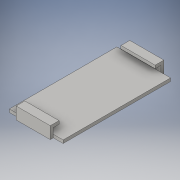
# Autodesk Inventor part: PanelHolder
Saved by Autodesk Inventor 2016 (Build 200138000, 138)
## iProperties
Created: 2016-08-20
Part Number: PanelHolder
Material: Generic
Document SubType Name: Modeling
Designer: yash
Density: 1 g/cm^3
Appearance: Default
Author: yash
Autodesk Inventor part; units mm, degrees
ref_plane "YZ Plane" through (0, 0, 0) normal (1, 0, 0) x (0, 1, 0)
ref_plane "XZ Plane" through (0, 0, 0) normal (0, 1, 0) x (-1, 0, 0)
ref_plane "XY Plane" through (0, 0, 0) normal (0, 0, 1) x (1, 0, 0)
sketch "Sketch1" plane through (0, 0, 0) normal (0, 1, 0) x (-1, 0, 0)
  line L0 (0, 0) -> (30, 0)
  line L1 (30, 0) -> (30, -60)
  line L2 (30, -60) -> (0, -60)
  line L3 (0, -60) -> (0, 0)
  dimension "d0" = 30
  dimension "d1" = 60
  constraints: 8 end point, 2 parallel, 1 horizontal, 1 perpendicular
  measures "d0" distance of L1.end L2.end
  measures "d1" distance of L0.end L1.end
extrude "Extrusion1" add sketch "Sketch1" along normal blind 1.7272
sketch "Sketch2" plane through (-30, 0, 0) normal (0, 0, 1) x (1, 0, 0)
  line L0 (30, 0) -> (0, 0) projected
  line L1 (5.475, 0) -> (24.525, 0)
  line L2 (24.525, 0) -> (24.525, 6.7272)
  line L3 (24.525, 6.7272) -> (5.475, 6.7272)
  line L4 (5.475, 6.7272) -> (5.475, 0)
  point P0 (15, 6.7272)
  point P1 (15, 0)
  dimension "d4" = 19.05
  dimension "d5" = 6.7272
  constraints: 8 end point, 2 midpoint, 2 parallel, 1 horizontal, 1 perpendicular, 1 point on line, 1 vertical alignment
  measures "d4" distance of L3.end L2.end
  measures "d5" distance of L2.end L1.end
extrude "Extrusion2" add sketch "Sketch2" along normal blind 1.7272
sketch "Sketch3" plane through (-30, 0, 0) normal (0, 0, -1) x (-1, 0, 0)
  line L0 (-24.525, 6.7272) -> (-5.475, 6.7272) projected
  line L1 (-5.475, 6.7272) -> (-5.475, 1.7272) projected
  line L2 (-24.525, 6.7272) -> (-5.475, 6.7272)
  line L3 (-5.475, 6.7272) -> (-5.475, 5)
  line L4 (-5.475, 5) -> (-24.525, 5)
  line L5 (-24.525, 5) -> (-24.525, 6.7272)
  point P0 (-30, 0)
  dimension "d8" = 1.7272
  constraints: 8 end point, 2 parallel, 1 horizontal, 1 perpendicular, 1 point on line
  measures "d8" distance of L2.end L3.end
extrude "Extrusion3" add sketch "Sketch3" along normal blind 3.175
sketch "Sketch4" plane through (0, 0, -60) normal (0, 0, -1) x (-1, 0, 0)
  line L0 (30, 0) -> (0, 0) projected
  line L1 (5.475, 6.7272) -> (24.525, 6.7272)
  line L2 (24.525, 6.7272) -> (24.525, 0)
  line L3 (24.525, 0) -> (5.475, 0)
  line L4 (5.475, 0) -> (5.475, 6.7272)
  line L5 (24.525, 6.7272) -> (5.475, 6.7272) projected
  point P0 (15, 6.7272)
  point P1 (15, 6.7272)
  dimension "d11" = 19.05
  dimension "d12" = 6.7272
  constraints: 8 end point, 2 midpoint, 2 parallel, 1 coincident, 1 horizontal, 1 perpendicular, 1 point on line
  measures "d11" distance of L1.start L1.end
  measures "d12" distance of L1.end L2.end
extrude "Extrusion4" add sketch "Sketch4" along normal blind 1.7272
sketch "Sketch5" plane through (0, 0, -60) normal (0, 0, 1) x (1, 0, 0)
  line L0 (-5.475, 6.7272) -> (-24.525, 6.7272) projected
  line L1 (-5.475, 1.7272) -> (-5.475, 6.7272) projected
  line L2 (-24.525, 6.7272) -> (-5.475, 6.7272)
  line L3 (-5.475, 6.7272) -> (-5.475, 5)
  line L4 (-5.475, 5) -> (-24.525, 5)
  line L5 (-24.525, 5) -> (-24.525, 6.7272)
  point P0 (0, 0)
  dimension "d15" = 1.7272
  constraints: 8 end point, 2 parallel, 1 horizontal, 1 perpendicular, 1 point on line
  measures "d15" distance of L2.end L3.end
extrude "Extrusion5" add sketch "Sketch5" along normal blind 3.175
body "Solid1"
